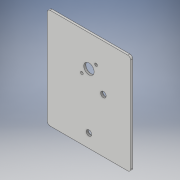
# Autodesk Inventor part: 板
Saved by Autodesk Inventor 2019 (Build 230136000, 136)
## iProperties
Created: 2020-09-28
Part Number: 板
Material: 一般
Document SubType Name: Modeling
Designer: zhept
Density: 1 g/cm^3
Appearance: 既定
Mass: 51.041 g
Surface Area: 359.608 cm^2
Volume: 51.041 cm^3
Author: zhept
Autodesk Inventor part; units mm, degrees
ref_plane "YZ Plane" through (0, 0, 0) normal (1, 0, 0) x (0, 1, 0)
ref_plane "XZ Plane" through (0, 0, 0) normal (0, 1, 0) x (-1, 0, 0)
ref_plane "XY Plane" through (0, 0, 0) normal (0, 0, 1) x (1, 0, 0)
sketch "スケッチ1" plane through (0, 0, 0) normal (0, 0, 1) x (1, 0, 0)
  circle A0 centre (0, 0) radius 21.2
  circle A1 centre (0, 0) radius 7.5
  circle A2 centre (0, 0) radius 30
  circle A3 centre (20.819222, -21.6) radius 22.5
  circle A4 centre (20.819222, -21.6) radius 14
  circle A5 centre (20.819222, -21.6) radius 62
  circle A6 centre (0, -80) radius 48
  circle A7 centre (0, -80) radius 50
  circle A8 centre (20.819222, -21.6) radius 4
  circle A9 centre (0, -80) radius 4
  dimension "d2" = 60
  dimension "d4" = 124
  dimension "d0" = 42.4
  dimension "d1" = 15
  dimension "d3" = 28
  dimension "d5" = 100
  dimension "d23" = 8
  dimension "d41" = 8
  constraints: 9 coincident, 8 centre point, 2 tangent, 6 other
  measures "d0" diameter of A0
  measures "d1" diameter of A1
  measures "d3" diameter of A4
  measures "d5" diameter of A7
  measures "d23" diameter of A8
  measures "d41" diameter of A9
sketch "スケッチ2" plane through (0, 0, 0) normal (0, 0, 1) x (1, 0, 0)
  line L0 (0, 0) -> (24.501973, 0) construction
  line L1 (0, 0) -> (12.5, 0) construction
  line L2 (0, 0) -> (10.253048, 10.253048)
  line L3 (0, 0) -> (14.5, 0) construction
  line L4 (10.253048, 10.253048) -> (-10.253048, -10.253048)
  circle A0 centre (10.253048, 10.253048) radius 2
  circle A1 centre (-10.253048, -10.253048) radius 2
  circle A2 centre (0, 0) radius 7.5
  line L5 (0, 0) -> (28.190779, 10.260604)
  line L6 (0, 0) -> (30, 0) construction
  line L7 (0, 0) -> (-28.190779, 10.260604)
  line L8 (0, 0) -> (30, 0) construction
  circle A3 centre (-28.190779, 10.260604) radius 2.5
  line L9 (0, 0) -> (0, 30)
  circle A4 centre (0, 30) radius 2.5
  circle A5 centre (28.190779, 10.260604) radius 2.5
  dimension "d9" = 14.5
  dimension "d10" = 45
  dimension "d11" = 29
  dimension "d12" = 4
  dimension "d13" = 4
  dimension "d14" = 15
  dimension "d15" = 30
  dimension "d16" = 20
  dimension "d17" = 30
  dimension "d18" = 160
  dimension "d19" = 5
  dimension "d20" = 30
  dimension "d21" = 5
  dimension "d22" = 5
  constraints: 20 end point, 6 centre point, 6 coincident, 5 horizontal, 3 equal length, 1 point on line, 1 vertical
  measures "d9" distance of L0.start L2.end
  measures "d10" angle of L3 L2
  measures "d11" distance of L2.end L4.end
  measures "d12" diameter of A0
  measures "d13" diameter of A1
  measures "d14" diameter of A2
  measures "d15" distance of L5.start L5.end
  measures "d16" angle of L6 L5
  measures "d17" distance of L5.start L7.end
  measures "d18" angle of L8 L7
  measures "d19" diameter of A3
  measures "d20" distance of L5.start L9.end
  measures "d21" diameter of A4
  measures "d22" diameter of A5
sketch "スケッチ3" plane through (0, 0, 0) normal (0, 0, 1) x (1, 0, 0)
  line L0 (60, -99.343647) -> (-60, -99.343647)
  line L1 (-60, -99.343647) -> (-60, 99.343647)
  line L2 (-60, 99.343647) -> (60, 99.343647)
  line L3 (60, 99.343647) -> (60, -99.343647)
  line L4 (60, -99.343647) -> (-60, 99.343647) construction
  line L5 (-60, -99.343647) -> (60, 99.343647) construction
  point P0 (0, 0)
  dimension "d25" = 120
  constraints: 12 end point, 2 midpoint, 2 parallel, 1 horizontal, 1 perpendicular
  measures "d25" distance of L0.start L0.end
extrude "押し出し1" add sketch "スケッチ3" against normal blind 3
sketch "スケッチ4" plane through (0, 0, 0) normal (0, 0, 1) x (1, 0, 0)
  line L0 (0, 45.071117) -> (68.359536, 45.071117)
  line L1 (68.359536, 45.071117) -> (-74.382402, 45.071117)
  line L2 (-74.382402, 45.071117) -> (108.165644, 45.071117)
  line L3 (108.165644, 45.071117) -> (108.165644, 129.415375)
  line L4 (108.165644, 129.415375) -> (-74.382402, 129.415375)
  line L5 (-74.382402, 129.415375) -> (-74.382402, 45.071117)
  point P0 (0, 0)
  constraints: 12 end point, 2 horizontal, 2 parallel, 1 perpendicular, 1 point on line
extrude "押し出し4" cut sketch "スケッチ4" against normal blind 10
fillet "フィレット1" radius 4 4 edges at (-60, 45.0711, -1.5) (60, 45.0711, -1.5) (-60, -99.3436, -1.5) (60, -99.3436, -1.5)
extrude "押し出し7" cut sketch "スケッチ1" against normal blind 10 contours A8 A2 | A2 A8 | A9 A5 | A5 A9
extrude "押し出し9" cut sketch "スケッチ2" against normal blind 4 contours L9 A2 L2 | L5 A2 L4 | L2 A2 L5 | L4 A2 L7 | L7 A2 L9 | A0 | A1
equation "\"d46\" = d12"
